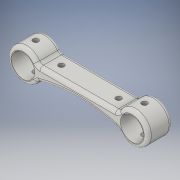
# Autodesk Inventor part: Carbon fibre tube original bracket 3.0
Saved by Autodesk Inventor 2016 (Build 200138000, 138)
## iProperties
Created: 2016-01-16
Part Number: Carbon fibre tube original bracket 3.0
Material: Generic
Document SubType Name: Modeling
Designer: Josiah Stark
Density: 1 g/cm^3
Appearance: Default
Author: Josiah Stark
Autodesk Inventor part; units mm, degrees
ref_plane "YZ Plane" through (0, 0, 0) normal (1, 0, 0) x (0, 1, 0)
sketch "Sketch1" plane through (0, 0, 0) normal (0, 0, 1) x (1, 0, 0)
  line L0 (28.2839, 10) -> (-28.2839, 10)
  circle A0 centre (-38.25, 5) radius 8.15
  circle A1 centre (38.25, 5) radius 8.15
  arc A2 (-28.2839, 10) -> (-28.2839, 0) centre (-38.25, 5) ccw
  arc A3 (28.2839, 0) -> (28.2839, 10) centre (38.25, 5) ccw
  arc A4 (28.2839, 0) -> (-28.2839, 0) centre (0, -97.5837) ccw
  point P0 (0, 0)
  dimension "d4" = 16.3
  dimension "d5" = 3
  dimension "d7" = 101.6
  constraints: 6 point on circle, 5 centre point, 2 end point
  measures "d4" diameter of A1
  measures "d5" radial gap between concentric circles of A0 A2
  measures "d7" radius of A4
extrude "Extrusion1" add sketch "Sketch1" along normal blind 17.5
ref_plane "Work Plane2" through (-28.2839, 17.62, 0) normal (0, 1, 0) x (1, 0, 0)
sketch "Sketch5" plane through (-28.2839, 17.62, 0) normal (0, 1, 0) x (1, 0, 0)
  line L0 (0, 0) -> (-21.1161, 0) projected
  line L1 (56.5679, -17.5) -> (77.6839, -17.5) projected
  line L2 (0, 0) -> (56.5679, 0)
  line L3 (56.5679, 0) -> (56.5679, -17.5)
  line L4 (56.5679, -17.5) -> (0, -17.5)
  line L5 (0, -17.5) -> (0, 0)
  line L6 (28.2839, 0) -> (28.2839, -17.5)
  line L7 (56.5679, -17.5) -> (0, -17.5) projected
  line L8 (28.2839, -8.75) -> (-8.0635, -8.75)
  line L9 (28.2839, -8.75) -> (64.6313, -8.75)
  circle A0 centre (-9.9685, -8.75) radius 1.905
  circle A1 centre (66.5363, -8.75) radius 1.905
  dimension "d39" = 3.81
  dimension "d40" = 3.81
  constraints: 14 end point, 3 horizontal, 2 horizontal alignment, 2 midpoint, 2 parallel, 1 perpendicular, 4 other
extrude "Extrusion4" cut sketch "Sketch5" against normal blind 25.4 contours A1 | A0
fillet "Fillet7" radius 3.175 4 edges at (-28.2839, 10, 8.75) (28.2839, 10, 8.75) (28.2839, 0, 8.75) (-28.2839, 0, 8.75)
fillet "Fillet8" radius 2.54 16 edges at (-27.9577, 10.3613, 17.5) (-49.3978, 4.7789, 17.5) (-28.058, -0.1481, 17.5) (0, 4.0163, 17.5) (28.058, -0.1481, 17.5) (49.3978, 4.7789, 17.5) (27.9577, 10.3613, 17.5) (0, 10, 17.5) (27.9577, 10.3613, 0) (49.3978, 4.7789, 0) (28.058, -0.1481, 0) (0, 4.0163, 0) (-28.058, -0.1481, 0) (-49.3978, 4.7789, 0) (-27.9577, 10.3613, 0) (0, 10, 0)
sketch "Sketch6" plane through (-26.4867, 10, 2.54) normal (0, 1, 0) x (1, 0, 0)
  line L0 (0, -12.42) -> (0, 0) projected
  line L1 (0, -6.21) -> (52.9734, -6.21)
  line L2 (52.9734, -6.21) -> (46.6234, -6.21)
  line L3 (0, -6.21) -> (6.35, -6.21)
  circle A0 centre (6.35, -6.21) radius 1.905
  circle A1 centre (46.6234, -6.21) radius 1.905
  point P0 (26.4867, 2.54)
  dimension "d45" = 6.35
  dimension "d46" = 6.35
  dimension "d47" = 3.81
  dimension "d48" = 3.81
  dimension "d57" = 40.2734
  constraints: 6 end point, 2 centre point, 2 coincident, 2 point on line, 1 horizontal, 1 midpoint
  measures "d45" distance of L1.end L2.end
  measures "d46" distance of L1.start L3.end
  measures "d47" diameter of A0
  measures "d48" diameter of A1
  measures "d57" distance of L2.end L3.end
extrude "Extrusion5" cut sketch "Sketch6" against normal blind 25.4
ref_plane "Work Plane3" through (-26.4867, -0.16, 2.54) normal (0, 1, 0) x (1, 0, 0)
sketch "Sketch7" plane through (-26.4867, -0.16, 2.54) normal (0, 1, 0) x (1, 0, 0)
  circle A0 centre (6.35, -6.21) radius 1.905 projected
  circle A1 centre (6.35, -6.21) radius 3.81
  circle A2 centre (46.6234, -6.21) radius 1.905 projected
  circle A3 centre (46.6234, -6.21) radius 3.81
  point P0 (26.4867, 2.54)
  dimension "d52" = 7.62
  dimension "d53" = 7.62
  constraints: 2 centre point, 2 coincident
  measures "d52" diameter of A1
  measures "d53" diameter of A3
extrude "Extrusion6" cut sketch "Sketch7" along normal blind 5.08
fillet "Fillet9" radius 1.27 4 edges at (-23.9459, 1.1541, 8.8274) (16.3273, 2.6958, 8.8216) (16.3267, 4.92, 8.75) (-23.9467, 4.92, 8.75)
body "Solid1"
